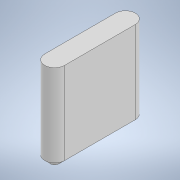
# Autodesk Inventor part: Contenedor anti-fuga (para imprimir en modo espiral)
Saved by Autodesk Inventor 2022 (Build 260153000, 153)
## iProperties
Created: 2022-02-11
Part Number: Contenedor anti-fuga (para imprimir en modo espiral)
Material: Generic
Document SubType Name: Modeling
Designer: juanp
Density: 1 g/cm^3
Appearance: Default
Author: juanp
Autodesk Inventor part; units mm, degrees
ref_plane "YZ Plane" through (0, 0, 0) normal (1, 0, 0) x (0, 1, 0)
ref_plane "XZ Plane" through (0, 0, 0) normal (0, 1, 0) x (-1, 0, 0)
ref_plane "XY Plane" through (0, 0, 0) normal (0, 0, 1) x (1, 0, 0)
sketch "Sketch1" plane through (0, 0, 0) normal (0, 1, 0) x (-1, 0, 0)
  line L0 (0, -19.4583) -> (0, 19.4583) construction
  line L1 (5.5417, -19.4583) -> (5.5417, 19.4583) construction
  line L2 (-5.5417, 19.4583) -> (-5.5417, -19.4583) construction
  arc A0 (-5.5417, -19.4583) -> (5.5417, -19.4583) centre (0, -19.4583) ccw construction
  arc A1 (5.5417, 19.4583) -> (-5.5417, 19.4583) centre (0, 19.4583) ccw construction
  line L3 (-5.4417, 19.4583) -> (-5.4417, -19.4583)
  arc A2 (-5.4417, -19.4583) -> (5.4417, -19.4583) centre (0, -19.4583) ccw
  line L4 (5.4417, -19.4583) -> (5.4417, 19.4583)
  arc A3 (5.4417, 19.4583) -> (-5.4417, 19.4583) centre (0, 19.4583) ccw
  point P0 (0, 0)
  dimension "d0" = 5.5417
  dimension "d1" = 38.9167
  dimension "d2" = 0.1
  constraints: 12 end point, 8 point on circle, 4 centre point, 4 tangent, 2 parallel, 1 midpoint, 1 vertical, 3 other
  measures "d0" radius of A1
  measures "d1" distance of L0.start L0.end
  measures "d2" radial gap between concentric circles of A1 A3
extrude "Extrusion1" add sketch "Sketch1" along normal blind 48.3333
chamfer "Chamfer1" distance 3 angle 45 4 edges at (5.4417, 0, 0) (0, 0, -24.9) (-5.4417, 0, 0) (0, 0, 24.9)
body "Solid1"
